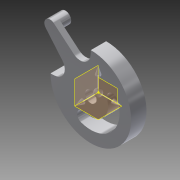
# Autodesk Inventor part: Geneva Drive
Saved by Autodesk Inventor 2018 (Build 220112000, 112)
## iProperties
Created: 2018-01-19
Part Number: Geneva Drive
Material: ABS Plastic
Document SubType Name: Sheet Metal
Designer: Rus
Density: 1.06 g/cm^3
Appearance: Smooth - White
Mass: 77.0184 g
Surface Area: 190.949 cm^2
Volume: 72.6589 cm^3
Sheet Metal Rule: Default
Author: Rus
Autodesk Inventor part; units mm, degrees
note: some values were not read from the file. Chosen so that the rebuilt part matches the saved one: second side of "Extrusion1".
ref_plane "YZ Plane" through (0, 0, 0) normal (1, 0, 0) x (0, 1, 0)
ref_plane "XZ Plane" through (0, 0, 0) normal (0, 1, 0) x (-1, 0, 0)
ref_plane "XY Plane" through (0, 0, 0) normal (0, 0, 1) x (1, 0, 0)
sketch "Sketch1" plane through (0, 0, 0) normal (0, 0, 1) x (1, 0, 0)
  line L0 (0, 0) -> (-89.8017, 0) construction
  line L1 (-89.8017, 0) -> (-44.9009, 44.9017) construction
  line L2 (-44.9009, 44.9017) -> (0, 0) construction
  arc A0 (-44.45, 0) -> (0.0009, 44.45) centre (0, 0) ccw
  line L3 (-44.45, 0) -> (-44.45, 44.4509) construction
  line L4 (-44.45, 44.4509) -> (-44.9009, 44.9017) construction
  circle A1 centre (-44.9009, 44.9017) radius 6.35
  arc A2 (-44.45, 0) -> (0.0009, 44.45) centre (-44.45, 44.4509) ccw
  point P0 (-6.7351, 6.7353)
  dimension "d8" = 89.8017
  dimension "d9" = 63.5
  dimension "d10" = 63.5
  dimension "d11" = 44.45
  dimension "d12" = 12.7
  constraints: 10 end point, 5 coincident, 4 point on circle, 3 centre point, 2 point on line, 1 collinear, 1 horizontal, 1 vertical
  measures "d8" distance of L0.start L0.end
  measures "d9" distance of L1.end L0.start
  measures "d10" distance of L0.end L1.end
  measures "d11" radius of A0
  measures "d12" diameter of A1
extrude "Extrusion1" add sketch "Sketch1" along normal blind 16.9333
sketch "Sketch21" plane through (-44.9009, 44.9017, 16.9333) normal (0, 0, 1) x (1, 0, 0)
  circle A0 centre (0, 0) radius 6.35 projected
  line L0 (4.0817, 4.8643) -> (26.0532, -13.5723)
  arc A1 (0.4509, -44.9017) -> (44.9017, -0.4517) centre (0.4509, -0.4509) ccw projected
  line L1 (-4.8644, -4.0817) -> (13.5718, -26.0535)
  circle A2 centre (0, 0) radius 6.35 projected
  line L2 (31.882, -31.8827) -> (26.0532, -13.5723) construction
  line L3 (31.882, -31.8827) -> (13.5718, -26.0535) construction
  arc A3 (6.4466, -44.4955) -> (13.5718, -26.0535) centre (4.9239, -33.3098) ccw
  arc A4 (26.0532, -13.5723) -> (44.4954, -6.4475) centre (33.3097, -4.9246) ccw
  line L4 (0, 0) -> (31.882, -31.8827) construction
  line L5 (13.5718, -26.0535) -> (15.941, -15.9413) construction
  line L6 (15.941, -15.9413) -> (26.0532, -13.5723) construction
  point P0 (44.9009, -44.9017)
  dimension "d85" = 10
  dimension "d86" = 11.2889
  constraints: 15 end point, 8 point on circle, 5 tangent, 2 centre point, 2 equal length, 1 equal radius, 1 midpoint, 2 other
  measures "d85" angle of L0 L1
  measures "d86" radius of A4
extrude "Extrusion18" add sketch "Sketch21" against normal blind 6.35 contours A0 L0 A4 A1 A3 L1
sketch "Sketch22" plane through (0, 0, 0) normal (0, 0, -1) x (-1, 0, 0)
  arc A0 (-17.9012, 6.5153) -> (6.5157, -17.9011) centre (0, 0) ccw
  arc A1 (-29.8353, 10.8589) -> (10.8594, -29.8351) centre (0, 0) ccw
  line L0 (10.8594, -29.8351) -> (6.5157, -17.9011)
  line L1 (-29.8353, 10.8589) -> (-17.9012, 6.5153)
  circle A2 centre (44.9009, 44.9017) radius 6.35 construction
  line L2 (6.5157, -17.9011) -> (44.9009, 44.9017) construction
  line L3 (44.9009, 44.9017) -> (-17.9012, 6.5153) construction
  arc A3 (-17.9012, 6.5153) -> (-29.8353, 10.8589) centre (-23.8683, 8.6871) ccw
  arc A4 (10.8594, -29.8351) -> (6.5157, -17.9011) centre (8.6875, -23.8681) ccw
  dimension "d89" = 19.05
  dimension "d90" = 12.7
  dimension "d91" = 130
  constraints: 8 end point, 8 point on circle, 4 centre point, 2 coincident, 2 point on line, 2 tangent, 1 equal length
  measures "d89" radius of A0
  measures "d90" radial gap between concentric circles of A0 A1
  measures "d91" angle of L0 L1
extrude "Extrusion19" cut sketch "Sketch22" against normal through all
sketch "Sketch23" plane through (0, 0, 0) normal (0, 0, -1) x (-1, 0, 0)
  circle A0 centre (0, 0) radius 6.35
  dimension "d94" = 12.7
  constraints: 1 centre point, 1 coincident
  measures "d94" diameter of A0
extrude "Extrusion20" cut sketch "Sketch23" against normal through all
body "Solid1"
